Autodesk Fusion 360 part; units mm, degrees
(part 8 of 14)
  line L4746 (-488.4472, -220.6625) -> (-493.9464, -211.1375)
  line L4747 (-493.9464, -230.1875) -> (-488.4472, -220.6625)
  line L4748 (-474.699, -200.025) -> (-485.6976, -200.025)
  line L4749 (-485.6976, -200.025) -> (-491.1968, -209.55)
  line L4750 (-491.1968, -209.55) -> (-485.6976, -219.075)
  line L4751 (-485.6976, -219.075) -> (-474.699, -219.075)
  line L4752 (-469.1998, -209.55) -> (-474.699, -200.025)
  line L4753 (-474.699, -219.075) -> (-469.1998, -209.55)
  line L4754 (-455.4516, -188.9125) -> (-466.4501, -188.9125)
  line L4755 (-466.4501, -188.9125) -> (-471.9494, -198.4375)
  line L4756 (-471.9494, -198.4375) -> (-466.4501, -207.9625)
  line L4757 (-466.4501, -207.9625) -> (-455.4516, -207.9625)
  line L4758 (-449.9524, -198.4375) -> (-455.4516, -188.9125)
  line L4759 (-455.4516, -207.9625) -> (-449.9524, -198.4375)
  line L4760 (-436.2042, -177.8) -> (-447.2027, -177.8)
  line L4761 (-447.2027, -177.8) -> (-452.702, -187.325)
  line L4762 (-452.702, -187.325) -> (-447.2027, -196.85)
  line L4763 (-447.2027, -196.85) -> (-436.2042, -196.85)
  line L4764 (-430.7049, -187.325) -> (-436.2042, -177.8)
  line L4765 (-436.2042, -196.85) -> (-430.7049, -187.325)
  line L4766 (-416.9568, -166.6875) -> (-427.9553, -166.6875)
  line L4767 (-427.9553, -166.6875) -> (-433.4546, -176.2125)
  line L4768 (-433.4546, -176.2125) -> (-427.9553, -185.7375)
  line L4769 (-427.9553, -185.7375) -> (-416.9568, -185.7375)
  line L4770 (-411.4575, -176.2125) -> (-416.9568, -166.6875)
  line L4771 (-416.9568, -185.7375) -> (-411.4575, -176.2125)
  line L4772 (-397.7094, -155.575) -> (-408.7079, -155.575)
  line L4773 (-408.7079, -155.575) -> (-414.2072, -165.1)
  line L4774 (-414.2072, -165.1) -> (-408.7079, -174.625)
  line L4775 (-408.7079, -174.625) -> (-397.7094, -174.625)
  line L4776 (-392.2101, -165.1) -> (-397.7094, -155.575)
  line L4777 (-397.7094, -174.625) -> (-392.2101, -165.1)
  line L4778 (-378.462, -144.4625) -> (-389.4605, -144.4625)
  line L4779 (-389.4605, -144.4625) -> (-394.9597, -153.9875)
  line L4780 (-394.9597, -153.9875) -> (-389.4605, -163.5125)
  line L4781 (-389.4605, -163.5125) -> (-378.462, -163.5125)
  line L4782 (-372.9627, -153.9875) -> (-378.462, -144.4625)
  line L4783 (-378.462, -163.5125) -> (-372.9627, -153.9875)
  line L4784 (-359.2145, -133.35) -> (-370.2131, -133.35)
  line L4785 (-370.2131, -133.35) -> (-375.7123, -142.875)
  line L4786 (-375.7123, -142.875) -> (-370.2131, -152.4)
  line L4787 (-370.2131, -152.4) -> (-359.2145, -152.4)
  line L4788 (-353.7153, -142.875) -> (-359.2145, -133.35)
  line L4789 (-359.2145, -152.4) -> (-353.7153, -142.875)
  line L4790 (-339.9671, -122.2375) -> (-350.9657, -122.2375)
  line L4791 (-350.9657, -122.2375) -> (-356.4649, -131.7625)
  line L4792 (-356.4649, -131.7625) -> (-350.9657, -141.2875)
  line L4793 (-350.9657, -141.2875) -> (-339.9671, -141.2875)
  line L4794 (-334.4679, -131.7625) -> (-339.9671, -122.2375)
  line L4795 (-339.9671, -141.2875) -> (-334.4679, -131.7625)
  line L4796 (-320.7197, -111.125) -> (-331.7182, -111.125)
  line L4797 (-331.7182, -111.125) -> (-337.2175, -120.65)
  line L4798 (-337.2175, -120.65) -> (-331.7182, -130.175)
  line L4799 (-331.7182, -130.175) -> (-320.7197, -130.175)
  line L4800 (-315.2205, -120.65) -> (-320.7197, -111.125)
  line L4801 (-320.7197, -130.175) -> (-315.2205, -120.65)
  line L4802 (-301.4723, -100.0125) -> (-312.4708, -100.0125)
  line L4803 (-312.4708, -100.0125) -> (-317.9701, -109.5375)
  line L4804 (-317.9701, -109.5375) -> (-312.4708, -119.0625)
  line L4805 (-312.4708, -119.0625) -> (-301.4723, -119.0625)
  line L4806 (-295.973, -109.5375) -> (-301.4723, -100.0125)
  line L4807 (-301.4723, -119.0625) -> (-295.973, -109.5375)
  line L4808 (-282.2249, -88.9) -> (-293.2234, -88.9)
  line L4809 (-293.2234, -88.9) -> (-298.7227, -98.425)
  line L4810 (-298.7227, -98.425) -> (-293.2234, -107.95)
  line L4811 (-293.2234, -107.95) -> (-282.2249, -107.95)
  line L4812 (-276.7256, -98.425) -> (-282.2249, -88.9)
  line L4813 (-282.2249, -107.95) -> (-276.7256, -98.425)
  line L4814 (-262.9775, -77.7875) -> (-273.976, -77.7875)
  line L4815 (-273.976, -77.7875) -> (-279.4753, -87.3125)
  line L4816 (-279.4753, -87.3125) -> (-273.976, -96.8375)
  line L4817 (-273.976, -96.8375) -> (-262.9775, -96.8375)
  line L4818 (-257.4782, -87.3125) -> (-262.9775, -77.7875)
  line L4819 (-262.9775, -96.8375) -> (-257.4782, -87.3125)
  line L4820 (-243.7301, -66.675) -> (-254.7286, -66.675)
  line L4821 (-254.7286, -66.675) -> (-260.2278, -76.2)
  line L4822 (-260.2278, -76.2) -> (-254.7286, -85.725)
  line L4823 (-254.7286, -85.725) -> (-243.7301, -85.725)
  line L4824 (-238.2308, -76.2) -> (-243.7301, -66.675)
  line L4825 (-243.7301, -85.725) -> (-238.2308, -76.2)
  line L4826 (-224.4826, -55.5625) -> (-235.4812, -55.5625)
  line L4827 (-235.4812, -55.5625) -> (-240.9804, -65.0875)
  line L4828 (-240.9804, -65.0875) -> (-235.4812, -74.6125)
  line L4829 (-235.4812, -74.6125) -> (-224.4826, -74.6125)
  line L4830 (-218.9834, -65.0875) -> (-224.4826, -55.5625)
  line L4831 (-224.4826, -74.6125) -> (-218.9834, -65.0875)
  line L4832 (-205.2352, -44.45) -> (-216.2337, -44.45)
  line L4833 (-216.2337, -44.45) -> (-221.733, -53.975)
  line L4834 (-221.733, -53.975) -> (-216.2337, -63.5)
  line L4835 (-216.2337, -63.5) -> (-205.2352, -63.5)
  line L4836 (-199.736, -53.975) -> (-205.2352, -44.45)
  line L4837 (-205.2352, -63.5) -> (-199.736, -53.975)
  line L4838 (-185.9878, -33.3375) -> (-196.9863, -33.3375)
  line L4839 (-196.9863, -33.3375) -> (-202.4856, -42.8625)
  line L4840 (-202.4856, -42.8625) -> (-196.9863, -52.3875)
  line L4841 (-196.9863, -52.3875) -> (-185.9878, -52.3875)
  line L4842 (-180.4886, -42.8625) -> (-185.9878, -33.3375)
  line L4843 (-185.9878, -52.3875) -> (-180.4886, -42.8625)
  line L4844 (-166.7404, -22.225) -> (-177.7389, -22.225)
  line L4845 (-177.7389, -22.225) -> (-183.2382, -31.75)
  line L4846 (-183.2382, -31.75) -> (-177.7389, -41.275)
  line L4847 (-177.7389, -41.275) -> (-166.7404, -41.275)
  line L4848 (-161.2411, -31.75) -> (-166.7404, -22.225)
  line L4849 (-166.7404, -41.275) -> (-161.2411, -31.75)
  line L4850 (-147.493, -11.1125) -> (-158.4915, -11.1125)
  line L4851 (-158.4915, -11.1125) -> (-163.9908, -20.6375)
  line L4852 (-163.9908, -20.6375) -> (-158.4915, -30.1625)
  line L4853 (-158.4915, -30.1625) -> (-147.493, -30.1625)
  line L4854 (-141.9937, -20.6375) -> (-147.493, -11.1125)
  line L4855 (-147.493, -30.1625) -> (-141.9937, -20.6375)
  line L4856 (-128.2456, 0) -> (-139.2441, 0)
  line L4857 (-139.2441, 0) -> (-144.7434, -9.525)
  line L4858 (-144.7434, -9.525) -> (-139.2441, -19.05)
  line L4859 (-139.2441, -19.05) -> (-128.2456, -19.05)
  line L4860 (-122.7463, -9.525) -> (-128.2456, 0)
  line L4861 (-128.2456, -19.05) -> (-122.7463, -9.525)
  line L4862 (-108.9982, 11.1125) -> (-119.9967, 11.1125)
  line L4863 (-119.9967, 11.1125) -> (-125.4959, 1.5875)
  line L4864 (-125.4959, 1.5875) -> (-119.9967, -7.9375)
  line L4865 (-119.9967, -7.9375) -> (-108.9982, -7.9375)
  line L4866 (-103.4989, 1.5875) -> (-108.9982, 11.1125)
  line L4867 (-108.9982, -7.9375) -> (-103.4989, 1.5875)
  line L4868 (-89.7507, 22.225) -> (-100.7493, 22.225)
  line L4869 (-100.7493, 22.225) -> (-106.2485, 12.7)
  line L4870 (-106.2485, 12.7) -> (-100.7493, 3.175)
  line L4871 (-100.7493, 3.175) -> (-89.7507, 3.175)
  line L4872 (-84.2515, 12.7) -> (-89.7507, 22.225)
  line L4873 (-89.7507, 3.175) -> (-84.2515, 12.7)
  line L4874 (-70.5033, 33.3375) -> (-81.5018, 33.3375)
  line L4875 (-81.5018, 33.3375) -> (-87.0011, 23.8125)
  line L4876 (-87.0011, 23.8125) -> (-81.5018, 14.2875)
  line L4877 (-81.5018, 14.2875) -> (-70.5033, 14.2875)
  line L4878 (-65.0041, 23.8125) -> (-70.5033, 33.3375)
  line L4879 (-70.5033, 14.2875) -> (-65.0041, 23.8125)
  line L4880 (-51.2559, 44.45) -> (-62.2544, 44.45)
  line L4881 (-62.2544, 44.45) -> (-67.7537, 34.925)
  line L4882 (-67.7537, 34.925) -> (-62.2544, 25.4)
  line L4883 (-62.2544, 25.4) -> (-51.2559, 25.4)
  line L4884 (-45.7566, 34.925) -> (-51.2559, 44.45)
  line L4885 (-51.2559, 25.4) -> (-45.7566, 34.925)
  line L4886 (-32.0085, 55.5625) -> (-43.007, 55.5625)
  line L4887 (-43.007, 55.5625) -> (-48.5063, 46.0375)
  line L4888 (-48.5063, 46.0375) -> (-43.007, 36.5125)
  line L4889 (-43.007, 36.5125) -> (-32.0085, 36.5125)
  line L4890 (-26.5092, 46.0375) -> (-32.0085, 55.5625)
  line L4891 (-32.0085, 36.5125) -> (-26.5092, 46.0375)
  line L4892 (-12.7611, 66.675) -> (-23.7596, 66.675)
  line L4893 (-23.7596, 66.675) -> (-29.2589, 57.15)
  line L4894 (-29.2589, 57.15) -> (-23.7596, 47.625)
  line L4895 (-23.7596, 47.625) -> (-12.7611, 47.625)
  line L4896 (-7.2618, 57.15) -> (-12.7611, 66.675)
  line L4897 (-12.7611, 47.625) -> (-7.2618, 57.15)
  line L4898 (6.4863, 77.7875) -> (-4.5122, 77.7875)
  line L4899 (-4.5122, 77.7875) -> (-10.0114, 68.2625)
  line L4900 (-10.0114, 68.2625) -> (-4.5122, 58.7375)
  line L4901 (-4.5122, 58.7375) -> (6.4863, 58.7375)
  line L4902 (11.9856, 68.2625) -> (6.4863, 77.7875)
  line L4903 (6.4863, 58.7375) -> (11.9856, 68.2625)
  line L4904 (25.7337, 88.9) -> (14.7352, 88.9)
  line L4905 (14.7352, 88.9) -> (9.236, 79.375)
  line L4906 (9.236, 79.375) -> (14.7352, 69.85)
  line L4907 (14.7352, 69.85) -> (25.7337, 69.85)
  line L4908 (31.233, 79.375) -> (25.7337, 88.9)
  line L4909 (25.7337, 69.85) -> (31.233, 79.375)
  line L4910 (44.9812, 100.0125) -> (33.9826, 100.0125)
  line L4911 (33.9826, 100.0125) -> (28.4834, 90.4875)
  line L4912 (28.4834, 90.4875) -> (33.9826, 80.9625)
  line L4913 (33.9826, 80.9625) -> (44.9812, 80.9625)
  line L4914 (50.4804, 90.4875) -> (44.9812, 100.0125)
  line L4915 (44.9812, 80.9625) -> (50.4804, 90.4875)
  line L4916 (64.2286, 111.125) -> (53.2301, 111.125)
  line L4917 (53.2301, 111.125) -> (47.7308, 101.6)
  line L4918 (47.7308, 101.6) -> (53.2301, 92.075)
  line L4919 (53.2301, 92.075) -> (64.2286, 92.075)
  line L4920 (69.7278, 101.6) -> (64.2286, 111.125)
  line L4921 (64.2286, 92.075) -> (69.7278, 101.6)
  line L4922 (83.476, 122.2375) -> (72.4775, 122.2375)
  line L4923 (72.4775, 122.2375) -> (66.9782, 112.7125)
  line L4924 (66.9782, 112.7125) -> (72.4775, 103.1875)
  line L4925 (72.4775, 103.1875) -> (83.476, 103.1875)
  line L4926 (88.9753, 112.7125) -> (83.476, 122.2375)
  line L4927 (83.476, 103.1875) -> (88.9753, 112.7125)
  line L4928 (102.7234, 133.35) -> (91.7249, 133.35)
  line L4929 (91.7249, 133.35) -> (86.2256, 123.825)
  line L4930 (86.2256, 123.825) -> (91.7249, 114.3)
  line L4931 (91.7249, 114.3) -> (102.7234, 114.3)
  line L4932 (108.2227, 123.825) -> (102.7234, 133.35)
  line L4933 (102.7234, 114.3) -> (108.2227, 123.825)
  line L4934 (121.9708, 144.4625) -> (110.9723, 144.4625)
  line L4935 (110.9723, 144.4625) -> (105.473, 134.9375)
  line L4936 (105.473, 134.9375) -> (110.9723, 125.4125)
  line L4937 (110.9723, 125.4125) -> (121.9708, 125.4125)
  line L4938 (127.4701, 134.9375) -> (121.9708, 144.4625)
  line L4939 (121.9708, 125.4125) -> (127.4701, 134.9375)
  line L4940 (141.2182, 155.575) -> (130.2197, 155.575)
  line L4941 (130.2197, 155.575) -> (124.7205, 146.05)
  line L4942 (124.7205, 146.05) -> (130.2197, 136.525)
  line L4943 (130.2197, 136.525) -> (141.2182, 136.525)
  line L4944 (146.7175, 146.05) -> (141.2182, 155.575)
  line L4945 (141.2182, 136.525) -> (146.7175, 146.05)
  line L4946 (160.4657, 166.6875) -> (149.4671, 166.6875)
  line L4947 (149.4671, 166.6875) -> (143.9679, 157.1625)
  line L4948 (143.9679, 157.1625) -> (149.4671, 147.6375)
  line L4949 (149.4671, 147.6375) -> (160.4657, 147.6375)
  line L4950 (165.9649, 157.1625) -> (160.4657, 166.6875)
  line L4951 (160.4657, 147.6375) -> (165.9649, 157.1625)
  line L4952 (179.7131, 177.8) -> (168.7145, 177.8)
  line L4953 (168.7145, 177.8) -> (163.2153, 168.275)
  line L4954 (163.2153, 168.275) -> (168.7145, 158.75)
  line L4955 (168.7145, 158.75) -> (179.7131, 158.75)
  line L4956 (185.2123, 168.275) -> (179.7131, 177.8)
  line L4957 (179.7131, 158.75) -> (185.2123, 168.275)
  line L4958 (198.9605, 188.9125) -> (187.962, 188.9125)
  line L4959 (187.962, 188.9125) -> (182.4627, 179.3875)
  line L4960 (182.4627, 179.3875) -> (187.962, 169.8625)
  line L4961 (187.962, 169.8625) -> (198.9605, 169.8625)
  line L4962 (204.4597, 179.3875) -> (198.9605, 188.9125)
  line L4963 (198.9605, 169.8625) -> (204.4597, 179.3875)
  line L4964 (218.2079, 200.025) -> (207.2094, 200.025)
  line L4965 (207.2094, 200.025) -> (201.7101, 190.5)
  line L4966 (201.7101, 190.5) -> (207.2094, 180.975)
  line L4967 (207.2094, 180.975) -> (218.2079, 180.975)
  line L4968 (223.7072, 190.5) -> (218.2079, 200.025)
  line L4969 (218.2079, 180.975) -> (223.7072, 190.5)
  line L4970 (237.4553, 211.1375) -> (226.4568, 211.1375)
  line L4971 (226.4568, 211.1375) -> (220.9575, 201.6125)
  line L4972 (220.9575, 201.6125) -> (226.4568, 192.0875)
  line L4973 (226.4568, 192.0875) -> (237.4553, 192.0875)
  line L4974 (242.9546, 201.6125) -> (237.4553, 211.1375)
  line L4975 (237.4553, 192.0875) -> (242.9546, 201.6125)
  line L4976 (256.7027, 222.25) -> (245.7042, 222.25)
  line L4977 (245.7042, 222.25) -> (240.2049, 212.725)
  line L4978 (240.2049, 212.725) -> (245.7042, 203.2)
  line L4979 (245.7042, 203.2) -> (256.7027, 203.2)
  line L4980 (262.202, 212.725) -> (256.7027, 222.25)
  line L4981 (256.7027, 203.2) -> (262.202, 212.725)
  line L4982 (275.9501, 233.3625) -> (264.9516, 233.3625)
  line L4983 (264.9516, 233.3625) -> (259.4524, 223.8375)
  line L4984 (259.4524, 223.8375) -> (264.9516, 214.3125)
  line L4985 (264.9516, 214.3125) -> (275.9501, 214.3125)
  line L4986 (281.4494, 223.8375) -> (275.9501, 233.3625)
  line L4987 (275.9501, 214.3125) -> (281.4494, 223.8375)
  line L4988 (295.1976, 244.475) -> (284.199, 244.475)
  line L4989 (284.199, 244.475) -> (278.6998, 234.95)
  line L4990 (278.6998, 234.95) -> (284.199, 225.425)
  line L4991 (284.199, 225.425) -> (295.1976, 225.425)
  line L4992 (300.6968, 234.95) -> (295.1976, 244.475)
  line L4993 (295.1976, 225.425) -> (300.6968, 234.95)
  line L4994 (314.445, 255.5875) -> (303.4464, 255.5875)
  line L4995 (303.4464, 255.5875) -> (297.9472, 246.0625)
  line L4996 (297.9472, 246.0625) -> (303.4464, 236.5375)
  line L4997 (303.4464, 236.5375) -> (314.445, 236.5375)
  line L4998 (319.9442, 246.0625) -> (314.445, 255.5875)
  line L4999 (314.445, 236.5375) -> (319.9442, 246.0625)
  line L5000 (333.6924, 266.7) -> (322.6939, 266.7)
  line L5001 (322.6939, 266.7) -> (317.1946, 257.175)
  line L5002 (317.1946, 257.175) -> (322.6939, 247.65)
  line L5003 (322.6939, 247.65) -> (333.6924, 247.65)
  line L5004 (339.1916, 257.175) -> (333.6924, 266.7)
  line L5005 (333.6924, 247.65) -> (339.1916, 257.175)
  line L5006 (352.9398, 277.8125) -> (341.9413, 277.8125)
  line L5007 (341.9413, 277.8125) -> (336.442, 268.2875)
  line L5008 (336.442, 268.2875) -> (341.9413, 258.7625)
  line L5009 (341.9413, 258.7625) -> (352.9398, 258.7625)
  line L5010 (358.4391, 268.2875) -> (352.9398, 277.8125)
  line L5011 (352.9398, 258.7625) -> (358.4391, 268.2875)
  line L5012 (372.1872, 288.925) -> (361.1887, 288.925)
  line L5013 (361.1887, 288.925) -> (355.6894, 279.4)
  line L5014 (355.6894, 279.4) -> (361.1887, 269.875)
  line L5015 (361.1887, 269.875) -> (372.1872, 269.875)
  line L5016 (377.6865, 279.4) -> (372.1872, 288.925)
  line L5017 (372.1872, 269.875) -> (377.6865, 279.4)
  line L5018 (391.4346, 300.0375) -> (380.4361, 300.0375)
  line L5019 (380.4361, 300.0375) -> (374.9368, 290.5125)
  line L5020 (374.9368, 290.5125) -> (380.4361, 280.9875)
  line L5021 (380.4361, 280.9875) -> (391.4346, 280.9875)
  line L5022 (396.9339, 290.5125) -> (391.4346, 300.0375)
  line L5023 (391.4346, 280.9875) -> (396.9339, 290.5125)
  line L5024 (410.682, 311.15) -> (399.6835, 311.15)
  line L5025 (399.6835, 311.15) -> (394.1843, 301.625)
  line L5026 (394.1843, 301.625) -> (399.6835, 292.1)
  line L5027 (399.6835, 292.1) -> (410.682, 292.1)
  line L5028 (416.1813, 301.625) -> (410.682, 311.15)
  line L5029 (410.682, 292.1) -> (416.1813, 301.625)
  line L5030 (429.9295, 322.2625) -> (418.9309, 322.2625)
  line L5031 (418.9309, 322.2625) -> (413.4317, 312.7375)
  line L5032 (413.4317, 312.7375) -> (418.9309, 303.2125)
  line L5033 (418.9309, 303.2125) -> (429.9295, 303.2125)
  line L5034 (435.4287, 312.7375) -> (429.9295, 322.2625)
  line L5035 (429.9295, 303.2125) -> (435.4287, 312.7375)
  line L5036 (449.1769, 333.375) -> (438.1783, 333.375)
  line L5037 (438.1783, 333.375) -> (432.6791, 323.85)
  line L5038 (432.6791, 323.85) -> (438.1783, 314.325)
  line L5039 (438.1783, 314.325) -> (449.1769, 314.325)
  line L5040 (454.6761, 323.85) -> (449.1769, 333.375)
  line L5041 (449.1769, 314.325) -> (454.6761, 323.85)
  line L5042 (468.4243, 344.4875) -> (457.4258, 344.4875)
  line L5043 (457.4258, 344.4875) -> (451.9265, 334.9625)
  line L5044 (451.9265, 334.9625) -> (457.4258, 325.4375)
  line L5045 (457.4258, 325.4375) -> (468.4243, 325.4375)
  line L5046 (473.9235, 334.9625) -> (468.4243, 344.4875)
  line L5047 (468.4243, 325.4375) -> (473.9235, 334.9625)
  line L5048 (487.6717, 355.6) -> (476.6732, 355.6)
  line L5049 (476.6732, 355.6) -> (471.1739, 346.075)
  line L5050 (471.1739, 346.075) -> (476.6732, 336.55)
  line L5051 (476.6732, 336.55) -> (487.6717, 336.55)
  line L5052 (493.171, 346.075) -> (487.6717, 355.6)
  line L5053 (487.6717, 336.55) -> (493.171, 346.075)
  line L5054 (506.9191, 366.7125) -> (495.9206, 366.7125)
  line L5055 (495.9206, 366.7125) -> (490.4213, 357.1875)
  line L5056 (490.4213, 357.1875) -> (495.9206, 347.6625)
  line L5057 (495.9206, 347.6625) -> (506.9191, 347.6625)
  line L5058 (512.4184, 357.1875) -> (506.9191, 366.7125)
  line L5059 (506.9191, 347.6625) -> (512.4184, 357.1875)
  line L5060 (-647.9258, -277.8125) -> (-658.9243, -277.8125)
  line L5061 (-658.9243, -277.8125) -> (-664.4235, -287.3375)
  line L5062 (-664.4235, -287.3375) -> (-658.9243, -296.8625)
  line L5063 (-658.9243, -296.8625) -> (-647.9258, -296.8625)
  line L5064 (-642.4265, -287.3375) -> (-647.9258, -277.8125)
  line L5065 (-647.9258, -296.8625) -> (-642.4265, -287.3375)
  line L5066 (-628.6783, -266.7) -> (-639.6769, -266.7)
  line L5067 (-639.6769, -266.7) -> (-645.1761, -276.225)
  line L5068 (-645.1761, -276.225) -> (-639.6769, -285.75)
  line L5069 (-639.6769, -285.75) -> (-628.6783, -285.75)
  line L5070 (-623.1791, -276.225) -> (-628.6783, -266.7)
  line L5071 (-628.6783, -285.75) -> (-623.1791, -276.225)
  line L5072 (-609.4309, -255.5875) -> (-620.4295, -255.5875)
  line L5073 (-620.4295, -255.5875) -> (-625.9287, -265.1125)
  line L5074 (-625.9287, -265.1125) -> (-620.4295, -274.6375)
  line L5075 (-620.4295, -274.6375) -> (-609.4309, -274.6375)
  line L5076 (-603.9317, -265.1125) -> (-609.4309, -255.5875)
  line L5077 (-609.4309, -274.6375) -> (-603.9317, -265.1125)
  line L5078 (-590.1835, -244.475) -> (-601.182, -244.475)
  line L5079 (-601.182, -244.475) -> (-606.6813, -254)
  line L5080 (-606.6813, -254) -> (-601.182, -263.525)
  line L5081 (-601.182, -263.525) -> (-590.1835, -263.525)
  line L5082 (-584.6843, -254) -> (-590.1835, -244.475)
  line L5083 (-590.1835, -263.525) -> (-584.6843, -254)
  line L5084 (-570.9361, -233.3625) -> (-581.9346, -233.3625)
  line L5085 (-581.9346, -233.3625) -> (-587.4339, -242.8875)
  line L5086 (-587.4339, -242.8875) -> (-581.9346, -252.4125)
  line L5087 (-581.9346, -252.4125) -> (-570.9361, -252.4125)
  line L5088 (-565.4368, -242.8875) -> (-570.9361, -233.3625)
  line L5089 (-570.9361, -252.4125) -> (-565.4368, -242.8875)
  line L5090 (-551.6887, -222.25) -> (-562.6872, -222.25)
  line L5091 (-562.6872, -222.25) -> (-568.1865, -231.775)
  line L5092 (-568.1865, -231.775) -> (-562.6872, -241.3)
  line L5093 (-562.6872, -241.3) -> (-551.6887, -241.3)
  line L5094 (-546.1894, -231.775) -> (-551.6887, -222.25)
  line L5095 (-551.6887, -241.3) -> (-546.1894, -231.775)
  line L5096 (-532.4413, -211.1375) -> (-543.4398, -211.1375)
  line L5097 (-543.4398, -211.1375) -> (-548.9391, -220.6625)
  line L5098 (-548.9391, -220.6625) -> (-543.4398, -230.1875)
  line L5099 (-543.4398, -230.1875) -> (-532.4413, -230.1875)
  line L5100 (-526.942, -220.6625) -> (-532.4413, -211.1375)
  line L5101 (-532.4413, -230.1875) -> (-526.942, -220.6625)
  line L5102 (-513.1939, -200.025) -> (-524.1924, -200.025)
  line L5103 (-524.1924, -200.025) -> (-529.6916, -209.55)
  line L5104 (-529.6916, -209.55) -> (-524.1924, -219.075)
  line L5105 (-524.1924, -219.075) -> (-513.1939, -219.075)
  line L5106 (-507.6946, -209.55) -> (-513.1939, -200.025)
  line L5107 (-513.1939, -219.075) -> (-507.6946, -209.55)
  line L5108 (-493.9464, -188.9125) -> (-504.945, -188.9125)
  line L5109 (-504.945, -188.9125) -> (-510.4442, -198.4375)
  line L5110 (-510.4442, -198.4375) -> (-504.945, -207.9625)
  line L5111 (-504.945, -207.9625) -> (-493.9464, -207.9625)
  line L5112 (-488.4472, -198.4375) -> (-493.9464, -188.9125)
  line L5113 (-493.9464, -207.9625) -> (-488.4472, -198.4375)
  line L5114 (-474.699, -177.8) -> (-485.6976, -177.8)
  line L5115 (-485.6976, -177.8) -> (-491.1968, -187.325)
  line L5116 (-491.1968, -187.325) -> (-485.6976, -196.85)
  line L5117 (-485.6976, -196.85) -> (-474.699, -196.85)
  line L5118 (-469.1998, -187.325) -> (-474.699, -177.8)
  line L5119 (-474.699, -196.85) -> (-469.1998, -187.325)
  line L5120 (-455.4516, -166.6875) -> (-466.4501, -166.6875)
  line L5121 (-466.4501, -166.6875) -> (-471.9494, -176.2125)
  line L5122 (-471.9494, -176.2125) -> (-466.4501, -185.7375)
  line L5123 (-466.4501, -185.7375) -> (-455.4516, -185.7375)
  line L5124 (-449.9524, -176.2125) -> (-455.4516, -166.6875)
  line L5125 (-455.4516, -185.7375) -> (-449.9524, -176.2125)
  line L5126 (-436.2042, -155.575) -> (-447.2027, -155.575)
  line L5127 (-447.2027, -155.575) -> (-452.702, -165.1)
  line L5128 (-452.702, -165.1) -> (-447.2027, -174.625)
  line L5129 (-447.2027, -174.625) -> (-436.2042, -174.625)
  line L5130 (-430.7049, -165.1) -> (-436.2042, -155.575)
  line L5131 (-436.2042, -174.625) -> (-430.7049, -165.1)
  line L5132 (-416.9568, -144.4625) -> (-427.9553, -144.4625)
  line L5133 (-427.9553, -144.4625) -> (-433.4546, -153.9875)
  line L5134 (-433.4546, -153.9875) -> (-427.9553, -163.5125)
  line L5135 (-427.9553, -163.5125) -> (-416.9568, -163.5125)
  line L5136 (-411.4575, -153.9875) -> (-416.9568, -144.4625)
  line L5137 (-416.9568, -163.5125) -> (-411.4575, -153.9875)
  line L5138 (-397.7094, -133.35) -> (-408.7079, -133.35)
  line L5139 (-408.7079, -133.35) -> (-414.2072, -142.875)
  line L5140 (-414.2072, -142.875) -> (-408.7079, -152.4)
  line L5141 (-408.7079, -152.4) -> (-397.7094, -152.4)
  line L5142 (-392.2101, -142.875) -> (-397.7094, -133.35)
  line L5143 (-397.7094, -152.4) -> (-392.2101, -142.875)
  line L5144 (-378.462, -122.2375) -> (-389.4605, -122.2375)
  line L5145 (-389.4605, -122.2375) -> (-394.9597, -131.7625)
  line L5146 (-394.9597, -131.7625) -> (-389.4605, -141.2875)
  line L5147 (-389.4605, -141.2875) -> (-378.462, -141.2875)
  line L5148 (-372.9627, -131.7625) -> (-378.462, -122.2375)
  line L5149 (-378.462, -141.2875) -> (-372.9627, -131.7625)
  line L5150 (-359.2145, -111.125) -> (-370.2131, -111.125)
  line L5151 (-370.2131, -111.125) -> (-375.7123, -120.65)
  line L5152 (-375.7123, -120.65) -> (-370.2131, -130.175)
  line L5153 (-370.2131, -130.175) -> (-359.2145, -130.175)
  line L5154 (-353.7153, -120.65) -> (-359.2145, -111.125)
  line L5155 (-359.2145, -130.175) -> (-353.7153, -120.65)
  line L5156 (-339.9671, -100.0125) -> (-350.9657, -100.0125)
  line L5157 (-350.9657, -100.0125) -> (-356.4649, -109.5375)
  line L5158 (-356.4649, -109.5375) -> (-350.9657, -119.0625)
  line L5159 (-350.9657, -119.0625) -> (-339.9671, -119.0625)
  line L5160 (-334.4679, -109.5375) -> (-339.9671, -100.0125)
  line L5161 (-339.9671, -119.0625) -> (-334.4679, -109.5375)
  line L5162 (-320.7197, -88.9) -> (-331.7182, -88.9)
  line L5163 (-331.7182, -88.9) -> (-337.2175, -98.425)
  line L5164 (-337.2175, -98.425) -> (-331.7182, -107.95)
  line L5165 (-331.7182, -107.95) -> (-320.7197, -107.95)
  line L5166 (-315.2205, -98.425) -> (-320.7197, -88.9)
  line L5167 (-320.7197, -107.95) -> (-315.2205, -98.425)
  line L5168 (-301.4723, -77.7875) -> (-312.4708, -77.7875)
  line L5169 (-312.4708, -77.7875) -> (-317.9701, -87.3125)
  line L5170 (-317.9701, -87.3125) -> (-312.4708, -96.8375)
  line L5171 (-312.4708, -96.8375) -> (-301.4723, -96.8375)
  line L5172 (-295.973, -87.3125) -> (-301.4723, -77.7875)
  line L5173 (-301.4723, -96.8375) -> (-295.973, -87.3125)
  line L5174 (-282.2249, -66.675) -> (-293.2234, -66.675)
  line L5175 (-293.2234, -66.675) -> (-298.7227, -76.2)
  line L5176 (-298.7227, -76.2) -> (-293.2234, -85.725)
  line L5177 (-293.2234, -85.725) -> (-282.2249, -85.725)
  line L5178 (-276.7256, -76.2) -> (-282.2249, -66.675)
  line L5179 (-282.2249, -85.725) -> (-276.7256, -76.2)
  line L5180 (-262.9775, -55.5625) -> (-273.976, -55.5625)
  line L5181 (-273.976, -55.5625) -> (-279.4753, -65.0875)
  line L5182 (-279.4753, -65.0875) -> (-273.976, -74.6125)
  line L5183 (-273.976, -74.6125) -> (-262.9775, -74.6125)
  line L5184 (-257.4782, -65.0875) -> (-262.9775, -55.5625)
  line L5185 (-262.9775, -74.6125) -> (-257.4782, -65.0875)
  line L5186 (-243.7301, -44.45) -> (-254.7286, -44.45)
  line L5187 (-254.7286, -44.45) -> (-260.2278, -53.975)
  line L5188 (-260.2278, -53.975) -> (-254.7286, -63.5)
  line L5189 (-254.7286, -63.5) -> (-243.7301, -63.5)
  line L5190 (-238.2308, -53.975) -> (-243.7301, -44.45)
  line L5191 (-243.7301, -63.5) -> (-238.2308, -53.975)
  line L5192 (-224.4826, -33.3375) -> (-235.4812, -33.3375)
  line L5193 (-235.4812, -33.3375) -> (-240.9804, -42.8625)
  line L5194 (-240.9804, -42.8625) -> (-235.4812, -52.3875)
  line L5195 (-235.4812, -52.3875) -> (-224.4826, -52.3875)
  line L5196 (-218.9834, -42.8625) -> (-224.4826, -33.3375)
  line L5197 (-224.4826, -52.3875) -> (-218.9834, -42.8625)
  line L5198 (-205.2352, -22.225) -> (-216.2337, -22.225)
  line L5199 (-216.2337, -22.225) -> (-221.733, -31.75)
  line L5200 (-221.733, -31.75) -> (-216.2337, -41.275)
  line L5201 (-216.2337, -41.275) -> (-205.2352, -41.275)
  line L5202 (-199.736, -31.75) -> (-205.2352, -22.225)
  line L5203 (-205.2352, -41.275) -> (-199.736, -31.75)
  line L5204 (-185.9878, -11.1125) -> (-196.9863, -11.1125)
  line L5205 (-196.9863, -11.1125) -> (-202.4856, -20.6375)
  line L5206 (-202.4856, -20.6375) -> (-196.9863, -30.1625)
  line L5207 (-196.9863, -30.1625) -> (-185.9878, -30.1625)
  line L5208 (-180.4886, -20.6375) -> (-185.9878, -11.1125)
  line L5209 (-185.9878, -30.1625) -> (-180.4886, -20.6375)
  line L5210 (-166.7404, 0) -> (-177.7389, 0)
  line L5211 (-177.7389, 0) -> (-183.2382, -9.525)
  line L5212 (-183.2382, -9.525) -> (-177.7389, -19.05)
  line L5213 (-177.7389, -19.05) -> (-166.7404, -19.05)
  line L5214 (-161.2411, -9.525) -> (-166.7404, 0)
  line L5215 (-166.7404, -19.05) -> (-161.2411, -9.525)
  line L5216 (-147.493, 11.1125) -> (-158.4915, 11.1125)
  line L5217 (-158.4915, 11.1125) -> (-163.9908, 1.5875)
  line L5218 (-163.9908, 1.5875) -> (-158.4915, -7.9375)
  line L5219 (-158.4915, -7.9375) -> (-147.493, -7.9375)
  line L5220 (-141.9937, 1.5875) -> (-147.493, 11.1125)
  line L5221 (-147.493, -7.9375) -> (-141.9937, 1.5875)
  line L5222 (-128.2456, 22.225) -> (-139.2441, 22.225)
  line L5223 (-139.2441, 22.225) -> (-144.7434, 12.7)
  line L5224 (-144.7434, 12.7) -> (-139.2441, 3.175)
  line L5225 (-139.2441, 3.175) -> (-128.2456, 3.175)
  line L5226 (-122.7463, 12.7) -> (-128.2456, 22.225)
  line L5227 (-128.2456, 3.175) -> (-122.7463, 12.7)
  line L5228 (-108.9982, 33.3375) -> (-119.9967, 33.3375)
  line L5229 (-119.9967, 33.3375) -> (-125.4959, 23.8125)
  line L5230 (-125.4959, 23.8125) -> (-119.9967, 14.2875)
  line L5231 (-119.9967, 14.2875) -> (-108.9982, 14.2875)
  line L5232 (-103.4989, 23.8125) -> (-108.9982, 33.3375)
  line L5233 (-108.9982, 14.2875) -> (-103.4989, 23.8125)
  line L5234 (-70.5033, 55.5625) -> (-81.5018, 55.5625)
  line L5235 (-81.5018, 55.5625) -> (-87.0011, 46.0375)
  line L5236 (-87.0011, 46.0375) -> (-81.5018, 36.5125)
  line L5237 (-81.5018, 36.5125) -> (-70.5033, 36.5125)
  line L5238 (-65.0041, 46.0375) -> (-70.5033, 55.5625)
  line L5239 (-70.5033, 36.5125) -> (-65.0041, 46.0375)
  line L5240 (-51.2559, 66.675) -> (-62.2544, 66.675)
  line L5241 (-62.2544, 66.675) -> (-67.7537, 57.15)
  line L5242 (-67.7537, 57.15) -> (-62.2544, 47.625)
  line L5243 (-62.2544, 47.625) -> (-51.2559, 47.625)
  line L5244 (-45.7566, 57.15) -> (-51.2559, 66.675)
  line L5245 (-51.2559, 47.625) -> (-45.7566, 57.15)
  line L5246 (-32.0085, 77.7875) -> (-43.007, 77.7875)
  line L5247 (-43.007, 77.7875) -> (-48.5063, 68.2625)
  line L5248 (-48.5063, 68.2625) -> (-43.007, 58.7375)
  line L5249 (-43.007, 58.7375) -> (-32.0085, 58.7375)
  line L5250 (-26.5092, 68.2625) -> (-32.0085, 77.7875)
  line L5251 (-32.0085, 58.7375) -> (-26.5092, 68.2625)
  line L5252 (-12.7611, 88.9) -> (-23.7596, 88.9)
  line L5253 (-23.7596, 88.9) -> (-29.2589, 79.375)
  line L5254 (-29.2589, 79.375) -> (-23.7596, 69.85)
  line L5255 (-23.7596, 69.85) -> (-12.7611, 69.85)
  line L5256 (-7.2618, 79.375) -> (-12.7611, 88.9)
  line L5257 (-12.7611, 69.85) -> (-7.2618, 79.375)
  line L5258 (6.4863, 100.0125) -> (-4.5122, 100.0125)
  line L5259 (-4.5122, 100.0125) -> (-10.0114, 90.4875)
  line L5260 (-10.0114, 90.4875) -> (-4.5122, 80.9625)
  line L5261 (-4.5122, 80.9625) -> (6.4863, 80.9625)
  line L5262 (11.9856, 90.4875) -> (6.4863, 100.0125)
  line L5263 (6.4863, 80.9625) -> (11.9856, 90.4875)
  line L5264 (25.7337, 111.125) -> (14.7352, 111.125)
  line L5265 (14.7352, 111.125) -> (9.236, 101.6)
  line L5266 (9.236, 101.6) -> (14.7352, 92.075)
  line L5267 (14.7352, 92.075) -> (25.7337, 92.075)
  line L5268 (31.233, 101.6) -> (25.7337, 111.125)
  line L5269 (25.7337, 92.075) -> (31.233, 101.6)
  line L5270 (44.9812, 122.2375) -> (33.9826, 122.2375)
  line L5271 (33.9826, 122.2375) -> (28.4834, 112.7125)
  line L5272 (28.4834, 112.7125) -> (33.9826, 103.1875)
  line L5273 (33.9826, 103.1875) -> (44.9812, 103.1875)
  line L5274 (50.4804, 112.7125) -> (44.9812, 122.2375)
  line L5275 (44.9812, 103.1875) -> (50.4804, 112.7125)
  line L5276 (64.2286, 133.35) -> (53.2301, 133.35)
  line L5277 (53.2301, 133.35) -> (47.7308, 123.825)
  line L5278 (47.7308, 123.825) -> (53.2301, 114.3)
  line L5279 (53.2301, 114.3) -> (64.2286, 114.3)
  line L5280 (69.7278, 123.825) -> (64.2286, 133.35)
  line L5281 (64.2286, 114.3) -> (69.7278, 123.825)
  line L5282 (83.476, 144.4625) -> (72.4775, 144.4625)
  line L5283 (72.4775, 144.4625) -> (66.9782, 134.9375)
  line L5284 (66.9782, 134.9375) -> (72.4775, 125.4125)
  line L5285 (72.4775, 125.4125) -> (83.476, 125.4125)
  line L5286 (88.9753, 134.9375) -> (83.476, 144.4625)
  line L5287 (83.476, 125.4125) -> (88.9753, 134.9375)
  line L5288 (102.7234, 155.575) -> (91.7249, 155.575)
  line L5289 (91.7249, 155.575) -> (86.2256, 146.05)
  line L5290 (86.2256, 146.05) -> (91.7249, 136.525)
  line L5291 (91.7249, 136.525) -> (102.7234, 136.525)
  line L5292 (108.2227, 146.05) -> (102.7234, 155.575)
  line L5293 (102.7234, 136.525) -> (108.2227, 146.05)
  line L5294 (121.9708, 166.6875) -> (110.9723, 166.6875)
  line L5295 (110.9723, 166.6875) -> (105.473, 157.1625)
  line L5296 (105.473, 157.1625) -> (110.9723, 147.6375)
  line L5297 (110.9723, 147.6375) -> (121.9708, 147.6375)
  line L5298 (127.4701, 157.1625) -> (121.9708, 166.6875)
  line L5299 (121.9708, 147.6375) -> (127.4701, 157.1625)
  line L5300 (141.2182, 177.8) -> (130.2197, 177.8)
  line L5301 (130.2197, 177.8) -> (124.7205, 168.275)
  line L5302 (124.7205, 168.275) -> (130.2197, 158.75)
  line L5303 (130.2197, 158.75) -> (141.2182, 158.75)
  line L5304 (146.7175, 168.275) -> (141.2182, 177.8)
  line L5305 (141.2182, 158.75) -> (146.7175, 168.275)
  line L5306 (160.4657, 188.9125) -> (149.4671, 188.9125)
  line L5307 (149.4671, 188.9125) -> (143.9679, 179.3875)
  line L5308 (143.9679, 179.3875) -> (149.4671, 169.8625)
  line L5309 (149.4671, 169.8625) -> (160.4657, 169.8625)
  line L5310 (165.9649, 179.3875) -> (160.4657, 188.9125)
  line L5311 (160.4657, 169.8625) -> (165.9649, 179.3875)
  line L5312 (179.7131, 200.025) -> (168.7145, 200.025)
  line L5313 (168.7145, 200.025) -> (163.2153, 190.5)
  line L5314 (163.2153, 190.5) -> (168.7145, 180.975)
  line L5315 (168.7145, 180.975) -> (179.7131, 180.975)
  line L5316 (185.2123, 190.5) -> (179.7131, 200.025)
  line L5317 (179.7131, 180.975) -> (185.2123, 190.5)
  line L5318 (198.9605, 211.1375) -> (187.962, 211.1375)
  line L5319 (187.962, 211.1375) -> (182.4627, 201.6125)
  line L5320 (182.4627, 201.6125) -> (187.962, 192.0875)
  line L5321 (187.962, 192.0875) -> (198.9605, 192.0875)
  line L5322 (204.4597, 201.6125) -> (198.9605, 211.1375)
  line L5323 (198.9605, 192.0875) -> (204.4597, 201.6125)
  line L5324 (218.2079, 222.25) -> (207.2094, 222.25)
  line L5325 (207.2094, 222.25) -> (201.7101, 212.725)
  line L5326 (201.7101, 212.725) -> (207.2094, 203.2)
  line L5327 (207.2094, 203.2) -> (218.2079, 203.2)
  line L5328 (223.7072, 212.725) -> (218.2079, 222.25)
  line L5329 (218.2079, 203.2) -> (223.7072, 212.725)
  line L5330 (237.4553, 233.3625) -> (226.4568, 233.3625)
  line L5331 (226.4568, 233.3625) -> (220.9575, 223.8375)
  line L5332 (220.9575, 223.8375) -> (226.4568, 214.3125)
  line L5333 (226.4568, 214.3125) -> (237.4553, 214.3125)
  line L5334 (242.9546, 223.8375) -> (237.4553, 233.3625)
  line L5335 (237.4553, 214.3125) -> (242.9546, 223.8375)
  line L5336 (256.7027, 244.475) -> (245.7042, 244.475)
  line L5337 (245.7042, 244.475) -> (240.2049, 234.95)
  line L5338 (240.2049, 234.95) -> (245.7042, 225.425)
  line L5339 (245.7042, 225.425) -> (256.7027, 225.425)
  line L5340 (262.202, 234.95) -> (256.7027, 244.475)
  line L5341 (256.7027, 225.425) -> (262.202, 234.95)
  line L5342 (275.9501, 255.5875) -> (264.9516, 255.5875)
  line L5343 (264.9516, 255.5875) -> (259.4524, 246.0625)
  line L5344 (259.4524, 246.0625) -> (264.9516, 236.5375)
  line L5345 (264.9516, 236.5375) -> (275.9501, 236.5375)
  line L5346 (281.4494, 246.0625) -> (275.9501, 255.5875)
  line L5347 (275.9501, 236.5375) -> (281.4494, 246.0625)
  line L5348 (295.1976, 266.7) -> (284.199, 266.7)
  line L5349 (284.199, 266.7) -> (278.6998, 257.175)
  line L5350 (278.6998, 257.175) -> (284.199, 247.65)
  line L5351 (284.199, 247.65) -> (295.1976, 247.65)
  line L5352 (300.6968, 257.175) -> (295.1976, 266.7)
  line L5353 (295.1976, 247.65) -> (300.6968, 257.175)
  line L5354 (314.445, 277.8125) -> (303.4464, 277.8125)
  line L5355 (303.4464, 277.8125) -> (297.9472, 268.2875)
  line L5356 (297.9472, 268.2875) -> (303.4464, 258.7625)
  line L5357 (303.4464, 258.7625) -> (314.445, 258.7625)
  line L5358 (319.9442, 268.2875) -> (314.445, 277.8125)
  line L5359 (314.445, 258.7625) -> (319.9442, 268.2875)
  line L5360 (333.6924, 288.925) -> (322.6939, 288.925)
  line L5361 (322.6939, 288.925) -> (317.1946, 279.4)
  line L5362 (317.1946, 279.4) -> (322.6939, 269.875)
  line L5363 (322.6939, 269.875) -> (333.6924, 269.875)
  line L5364 (339.1916, 279.4) -> (333.6924, 288.925)
  line L5365 (333.6924, 269.875) -> (339.1916, 279.4)
  line L5366 (352.9398, 300.0375) -> (341.9413, 300.0375)
  line L5367 (341.9413, 300.0375) -> (336.442, 290.5125)
  line L5368 (336.442, 290.5125) -> (341.9413, 280.9875)
  line L5369 (341.9413, 280.9875) -> (352.9398, 280.9875)
  line L5370 (358.4391, 290.5125) -> (352.9398, 300.0375)
  line L5371 (352.9398, 280.9875) -> (358.4391, 290.5125)
  line L5372 (372.1872, 311.15) -> (361.1887, 311.15)
  line L5373 (361.1887, 311.15) -> (355.6894, 301.625)
  line L5374 (355.6894, 301.625) -> (361.1887, 292.1)
  line L5375 (361.1887, 292.1) -> (372.1872, 292.1)
  line L5376 (377.6865, 301.625) -> (372.1872, 311.15)
  line L5377 (372.1872, 292.1) -> (377.6865, 301.625)
  line L5378 (391.4346, 322.2625) -> (380.4361, 322.2625)
  line L5379 (380.4361, 322.2625) -> (374.9368, 312.7375)
  line L5380 (374.9368, 312.7375) -> (380.4361, 303.2125)
  line L5381 (380.4361, 303.2125) -> (391.4346, 303.2125)
  line L5382 (396.9339, 312.7375) -> (391.4346, 322.2625)
  line L5383 (391.4346, 303.2125) -> (396.9339, 312.7375)
  line L5384 (410.682, 333.375) -> (399.6835, 333.375)
  line L5385 (399.6835, 333.375) -> (394.1843, 323.85)
  line L5386 (394.1843, 323.85) -> (399.6835, 314.325)
  line L5387 (399.6835, 314.325) -> (410.682, 314.325)
  line L5388 (416.1813, 323.85) -> (410.682, 333.375)
  line L5389 (410.682, 314.325) -> (416.1813, 323.85)
  line L5390 (429.9295, 344.4875) -> (418.9309, 344.4875)
  line L5391 (418.9309, 344.4875) -> (413.4317, 334.9625)
  line L5392 (413.4317, 334.9625) -> (418.9309, 325.4375)
  line L5393 (418.9309, 325.4375) -> (429.9295, 325.4375)
  line L5394 (435.4287, 334.9625) -> (429.9295, 344.4875)
  line L5395 (429.9295, 325.4375) -> (435.4287, 334.9625)
  line L5396 (449.1769, 355.6) -> (438.1783, 355.6)
  line L5397 (438.1783, 355.6) -> (432.6791, 346.075)
  line L5398 (432.6791, 346.075) -> (438.1783, 336.55)
  line L5399 (438.1783, 336.55) -> (449.1769, 336.55)
  line L5400 (454.6761, 346.075) -> (449.1769, 355.6)
  line L5401 (449.1769, 336.55) -> (454.6761, 346.075)
  line L5402 (468.4243, 366.7125) -> (457.4258, 366.7125)
  line L5403 (457.4258, 366.7125) -> (451.9265, 357.1875)
  line L5404 (451.9265, 357.1875) -> (457.4258, 347.6625)
  line L5405 (457.4258, 347.6625) -> (468.4243, 347.6625)
  line L5406 (473.9235, 357.1875) -> (468.4243, 366.7125)
  line L5407 (468.4243, 347.6625) -> (473.9235, 357.1875)
  line L5408 (487.6717, 377.825) -> (476.6732, 377.825)
  line L5409 (476.6732, 377.825) -> (471.1739, 368.3)
  line L5410 (471.1739, 368.3) -> (476.6732, 358.775)
  line L5411 (476.6732, 358.775) -> (487.6717, 358.775)
  line L5412 (493.171, 368.3) -> (487.6717, 377.825)
  line L5413 (487.6717, 358.775) -> (493.171, 368.3)
  line L5414 (-667.1732, -266.7) -> (-678.1717, -266.7)
  line L5415 (-678.1717, -266.7) -> (-683.671, -276.225)
  line L5416 (-683.671, -276.225) -> (-678.1717, -285.75)
  line L5417 (-678.1717, -285.75) -> (-667.1732, -285.75)
  line L5418 (-661.6739, -276.225) -> (-667.1732, -266.7)
  line L5419 (-667.1732, -285.75) -> (-661.6739, -276.225)
  line L5420 (-647.9258, -255.5875) -> (-658.9243, -255.5875)
  line L5421 (-658.9243, -255.5875) -> (-664.4235, -265.1125)
  line L5422 (-664.4235, -265.1125) -> (-658.9243, -274.6375)
  line L5423 (-658.9243, -274.6375) -> (-647.9258, -274.6375)
  line L5424 (-642.4265, -265.1125) -> (-647.9258, -255.5875)
  line L5425 (-647.9258, -274.6375) -> (-642.4265, -265.1125)
  line L5426 (-628.6783, -244.475) -> (-639.6769, -244.475)
  line L5427 (-639.6769, -244.475) -> (-645.1761, -254)
  line L5428 (-645.1761, -254) -> (-639.6769, -263.525)
  line L5429 (-639.6769, -263.525) -> (-628.6783, -263.525)
  line L5430 (-623.1791, -254) -> (-628.6783, -244.475)
  line L5431 (-628.6783, -263.525) -> (-623.1791, -254)
  line L5432 (-609.4309, -233.3625) -> (-620.4295, -233.3625)
  line L5433 (-620.4295, -233.3625) -> (-625.9287, -242.8875)
  line L5434 (-625.9287, -242.8875) -> (-620.4295, -252.4125)
  line L5435 (-620.4295, -252.4125) -> (-609.4309, -252.4125)
  line L5436 (-603.9317, -242.8875) -> (-609.4309, -233.3625)
  line L5437 (-609.4309, -252.4125) -> (-603.9317, -242.8875)
  line L5438 (-590.1835, -222.25) -> (-601.182, -222.25)
  line L5439 (-601.182, -222.25) -> (-606.6813, -231.775)
  line L5440 (-606.6813, -231.775) -> (-601.182, -241.3)
  line L5441 (-601.182, -241.3) -> (-590.1835, -241.3)
  line L5442 (-584.6843, -231.775) -> (-590.1835, -222.25)
  line L5443 (-590.1835, -241.3) -> (-584.6843, -231.775)
  line L5444 (-570.9361, -211.1375) -> (-581.9346, -211.1375)
  line L5445 (-581.9346, -211.1375) -> (-587.4339, -220.6625)
  line L5446 (-587.4339, -220.6625) -> (-581.9346, -230.1875)
  line L5447 (-581.9346, -230.1875) -> (-570.9361, -230.1875)
  line L5448 (-565.4368, -220.6625) -> (-570.9361, -211.1375)
  line L5449 (-570.9361, -230.1875) -> (-565.4368, -220.6625)
  line L5450 (-551.6887, -200.025) -> (-562.6872, -200.025)
  line L5451 (-562.6872, -200.025) -> (-568.1865, -209.55)
  line L5452 (-568.1865, -209.55) -> (-562.6872, -219.075)
  line L5453 (-562.6872, -219.075) -> (-551.6887, -219.075)
  line L5454 (-546.1894, -209.55) -> (-551.6887, -200.025)
  line L5455 (-551.6887, -219.075) -> (-546.1894, -209.55)
  line L5456 (-532.4413, -188.9125) -> (-543.4398, -188.9125)
  line L5457 (-543.4398, -188.9125) -> (-548.9391, -198.4375)
  line L5458 (-548.9391, -198.4375) -> (-543.4398, -207.9625)
  line L5459 (-543.4398, -207.9625) -> (-532.4413, -207.9625)
  line L5460 (-526.942, -198.4375) -> (-532.4413, -188.9125)
  line L5461 (-532.4413, -207.9625) -> (-526.942, -198.4375)
  line L5462 (-513.1939, -177.8) -> (-524.1924, -177.8)
  line L5463 (-524.1924, -177.8) -> (-529.6916, -187.325)
  line L5464 (-529.6916, -187.325) -> (-524.1924, -196.85)
  line L5465 (-524.1924, -196.85) -> (-513.1939, -196.85)
  line L5466 (-507.6946, -187.325) -> (-513.1939, -177.8)
  line L5467 (-513.1939, -196.85) -> (-507.6946, -187.325)
  line L5468 (-493.9464, -166.6875) -> (-504.945, -166.6875)
  line L5469 (-504.945, -166.6875) -> (-510.4442, -176.2125)
  line L5470 (-510.4442, -176.2125) -> (-504.945, -185.7375)
  line L5471 (-504.945, -185.7375) -> (-493.9464, -185.7375)
  line L5472 (-488.4472, -176.2125) -> (-493.9464, -166.6875)
  line L5473 (-493.9464, -185.7375) -> (-488.4472, -176.2125)
  line L5474 (-474.699, -155.575) -> (-485.6976, -155.575)
  line L5475 (-485.6976, -155.575) -> (-491.1968, -165.1)
  line L5476 (-491.1968, -165.1) -> (-485.6976, -174.625)
  line L5477 (-485.6976, -174.625) -> (-474.699, -174.625)
  line L5478 (-469.1998, -165.1) -> (-474.699, -155.575)
  line L5479 (-474.699, -174.625) -> (-469.1998, -165.1)
  line L5480 (-455.4516, -144.4625) -> (-466.4501, -144.4625)
  line L5481 (-466.4501, -144.4625) -> (-471.9494, -153.9875)
  line L5482 (-471.9494, -153.9875) -> (-466.4501, -163.5125)
  line L5483 (-466.4501, -163.5125) -> (-455.4516, -163.5125)
  line L5484 (-449.9524, -153.9875) -> (-455.4516, -144.4625)
  line L5485 (-455.4516, -163.5125) -> (-449.9524, -153.9875)
  line L5486 (-436.2042, -133.35) -> (-447.2027, -133.35)
  line L5487 (-447.2027, -133.35) -> (-452.702, -142.875)
  line L5488 (-452.702, -142.875) -> (-447.2027, -152.4)
  line L5489 (-447.2027, -152.4) -> (-436.2042, -152.4)
  line L5490 (-430.7049, -142.875) -> (-436.2042, -133.35)
  line L5491 (-436.2042, -152.4) -> (-430.7049, -142.875)
  line L5492 (-416.9568, -122.2375) -> (-427.9553, -122.2375)
  line L5493 (-427.9553, -122.2375) -> (-433.4546, -131.7625)
  line L5494 (-433.4546, -131.7625) -> (-427.9553, -141.2875)
  line L5495 (-427.9553, -141.2875) -> (-416.9568, -141.2875)
  line L5496 (-411.4575, -131.7625) -> (-416.9568, -122.2375)
  line L5497 (-416.9568, -141.2875) -> (-411.4575, -131.7625)
  line L5498 (-397.7094, -111.125) -> (-408.7079, -111.125)
  line L5499 (-408.7079, -111.125) -> (-414.2072, -120.65)
  line L5500 (-414.2072, -120.65) -> (-408.7079, -130.175)
  line L5501 (-408.7079, -130.175) -> (-397.7094, -130.175)
  line L5502 (-392.2101, -120.65) -> (-397.7094, -111.125)
  line L5503 (-397.7094, -130.175) -> (-392.2101, -120.65)
  line L5504 (-378.462, -100.0125) -> (-389.4605, -100.0125)
  line L5505 (-389.4605, -100.0125) -> (-394.9597, -109.5375)
  line L5506 (-394.9597, -109.5375) -> (-389.4605, -119.0625)
  line L5507 (-389.4605, -119.0625) -> (-378.462, -119.0625)
  line L5508 (-372.9627, -109.5375) -> (-378.462, -100.0125)
  line L5509 (-378.462, -119.0625) -> (-372.9627, -109.5375)
  line L5510 (-359.2145, -88.9) -> (-370.2131, -88.9)
  line L5511 (-370.2131, -88.9) -> (-375.7123, -98.425)
  line L5512 (-375.7123, -98.425) -> (-370.2131, -107.95)
  line L5513 (-370.2131, -107.95) -> (-359.2145, -107.95)
  line L5514 (-353.7153, -98.425) -> (-359.2145, -88.9)
  line L5515 (-359.2145, -107.95) -> (-353.7153, -98.425)
  line L5516 (-339.9671, -77.7875) -> (-350.9657, -77.7875)
  line L5517 (-350.9657, -77.7875) -> (-356.4649, -87.3125)
  line L5518 (-356.4649, -87.3125) -> (-350.9657, -96.8375)
  line L5519 (-350.9657, -96.8375) -> (-339.9671, -96.8375)
  line L5520 (-334.4679, -87.3125) -> (-339.9671, -77.7875)
  line L5521 (-339.9671, -96.8375) -> (-334.4679, -87.3125)
  line L5522 (-320.7197, -66.675) -> (-331.7182, -66.675)
  line L5523 (-331.7182, -66.675) -> (-337.2175, -76.2)
  line L5524 (-337.2175, -76.2) -> (-331.7182, -85.725)
  line L5525 (-331.7182, -85.725) -> (-320.7197, -85.725)
  line L5526 (-315.2205, -76.2) -> (-320.7197, -66.675)
  line L5527 (-320.7197, -85.725) -> (-315.2205, -76.2)
  line L5528 (-301.4723, -55.5625) -> (-312.4708, -55.5625)
  line L5529 (-312.4708, -55.5625) -> (-317.9701, -65.0875)
  line L5530 (-317.9701, -65.0875) -> (-312.4708, -74.6125)
  line L5531 (-312.4708, -74.6125) -> (-301.4723, -74.6125)
  line L5532 (-295.973, -65.0875) -> (-301.4723, -55.5625)
  line L5533 (-301.4723, -74.6125) -> (-295.973, -65.0875)
  line L5534 (-282.2249, -44.45) -> (-293.2234, -44.45)
  line L5535 (-293.2234, -44.45) -> (-298.7227, -53.975)
  line L5536 (-298.7227, -53.975) -> (-293.2234, -63.5)
  line L5537 (-293.2234, -63.5) -> (-282.2249, -63.5)
  line L5538 (-276.7256, -53.975) -> (-282.2249, -44.45)
  line L5539 (-282.2249, -63.5) -> (-276.7256, -53.975)
  line L5540 (-262.9775, -33.3375) -> (-273.976, -33.3375)
  line L5541 (-273.976, -33.3375) -> (-279.4753, -42.8625)
  line L5542 (-279.4753, -42.8625) -> (-273.976, -52.3875)
  line L5543 (-273.976, -52.3875) -> (-262.9775, -52.3875)
  line L5544 (-257.4782, -42.8625) -> (-262.9775, -33.3375)
  line L5545 (-262.9775, -52.3875) -> (-257.4782, -42.8625)
  line L5546 (-243.7301, -22.225) -> (-254.7286, -22.225)
  line L5547 (-254.7286, -22.225) -> (-260.2278, -31.75)
  line L5548 (-260.2278, -31.75) -> (-254.7286, -41.275)
  line L5549 (-254.7286, -41.275) -> (-243.7301, -41.275)
  line L5550 (-238.2308, -31.75) -> (-243.7301, -22.225)
  line L5551 (-243.7301, -41.275) -> (-238.2308, -31.75)
  line L5552 (-224.4826, -11.1125) -> (-235.4812, -11.1125)
  line L5553 (-235.4812, -11.1125) -> (-240.9804, -20.6375)
  line L5554 (-240.9804, -20.6375) -> (-235.4812, -30.1625)
  line L5555 (-235.4812, -30.1625) -> (-224.4826, -30.1625)
  line L5556 (-218.9834, -20.6375) -> (-224.4826, -11.1125)
  line L5557 (-224.4826, -30.1625) -> (-218.9834, -20.6375)
  line L5558 (-205.2352, 0) -> (-216.2337, 0)
  line L5559 (-216.2337, 0) -> (-221.733, -9.525)
  line L5560 (-221.733, -9.525) -> (-216.2337, -19.05)
  line L5561 (-216.2337, -19.05) -> (-205.2352, -19.05)
  line L5562 (-199.736, -9.525) -> (-205.2352, 0)
  line L5563 (-205.2352, -19.05) -> (-199.736, -9.525)
  line L5564 (-185.9878, 11.1125) -> (-196.9863, 11.1125)
  line L5565 (-196.9863, 11.1125) -> (-202.4856, 1.5875)
  line L5566 (-202.4856, 1.5875) -> (-196.9863, -7.9375)
  line L5567 (-196.9863, -7.9375) -> (-185.9878, -7.9375)
  line L5568 (-180.4886, 1.5875) -> (-185.9878, 11.1125)
  line L5569 (-185.9878, -7.9375) -> (-180.4886, 1.5875)
  line L5570 (-166.7404, 22.225) -> (-177.7389, 22.225)
  line L5571 (-177.7389, 22.225) -> (-183.2382, 12.7)
  line L5572 (-183.2382, 12.7) -> (-177.7389, 3.175)
  line L5573 (-177.7389, 3.175) -> (-166.7404, 3.175)
  line L5574 (-161.2411, 12.7) -> (-166.7404, 22.225)
  line L5575 (-166.7404, 3.175) -> (-161.2411, 12.7)
  line L5576 (-147.493, 33.3375) -> (-158.4915, 33.3375)
  line L5577 (-158.4915, 33.3375) -> (-163.9908, 23.8125)
  line L5578 (-163.9908, 23.8125) -> (-158.4915, 14.2875)
  line L5579 (-158.4915, 14.2875) -> (-147.493, 14.2875)
  line L5580 (-141.9937, 23.8125) -> (-147.493, 33.3375)
  line L5581 (-147.493, 14.2875) -> (-141.9937, 23.8125)
  line L5582 (-128.2456, 44.45) -> (-139.2441, 44.45)
  line L5583 (-139.2441, 44.45) -> (-144.7434, 34.925)
  line L5584 (-144.7434, 34.925) -> (-139.2441, 25.4)
  line L5585 (-139.2441, 25.4) -> (-128.2456, 25.4)
  line L5586 (-122.7463, 34.925) -> (-128.2456, 44.45)
  line L5587 (-128.2456, 25.4) -> (-122.7463, 34.925)
  line L5588 (-108.9982, 55.5625) -> (-119.9967, 55.5625)
  line L5589 (-119.9967, 55.5625) -> (-125.4959, 46.0375)
  line L5590 (-125.4959, 46.0375) -> (-119.9967, 36.5125)
  line L5591 (-119.9967, 36.5125) -> (-108.9982, 36.5125)
  line L5592 (-103.4989, 46.0375) -> (-108.9982, 55.5625)
  line L5593 (-108.9982, 36.5125) -> (-103.4989, 46.0375)
  line L5594 (-89.7507, 66.675) -> (-100.7493, 66.675)
  line L5595 (-100.7493, 66.675) -> (-106.2485, 57.15)
  line L5596 (-106.2485, 57.15) -> (-100.7493, 47.625)
  line L5597 (-100.7493, 47.625) -> (-89.7507, 47.625)
  line L5598 (-84.2515, 57.15) -> (-89.7507, 66.675)
  line L5599 (-89.7507, 47.625) -> (-84.2515, 57.15)
  line L5600 (-70.5033, 77.7875) -> (-81.5018, 77.7875)
  line L5601 (-81.5018, 77.7875) -> (-87.0011, 68.2625)
  line L5602 (-87.0011, 68.2625) -> (-81.5018, 58.7375)
  line L5603 (-81.5018, 58.7375) -> (-70.5033, 58.7375)
  line L5604 (-65.0041, 68.2625) -> (-70.5033, 77.7875)
  line L5605 (-70.5033, 58.7375) -> (-65.0041, 68.2625)
  line L5606 (-51.2559, 88.9) -> (-62.2544, 88.9)
  line L5607 (-62.2544, 88.9) -> (-67.7537, 79.375)
  line L5608 (-67.7537, 79.375) -> (-62.2544, 69.85)
  line L5609 (-62.2544, 69.85) -> (-51.2559, 69.85)
  line L5610 (-45.7566, 79.375) -> (-51.2559, 88.9)
  line L5611 (-51.2559, 69.85) -> (-45.7566, 79.375)
  line L5612 (-32.0085, 100.0125) -> (-43.007, 100.0125)
  line L5613 (-43.007, 100.0125) -> (-48.5063, 90.4875)
  line L5614 (-48.5063, 90.4875) -> (-43.007, 80.9625)
  line L5615 (-43.007, 80.9625) -> (-32.0085, 80.9625)
  line L5616 (-26.5092, 90.4875) -> (-32.0085, 100.0125)
  line L5617 (-32.0085, 80.9625) -> (-26.5092, 90.4875)
  line L5618 (-12.7611, 111.125) -> (-23.7596, 111.125)